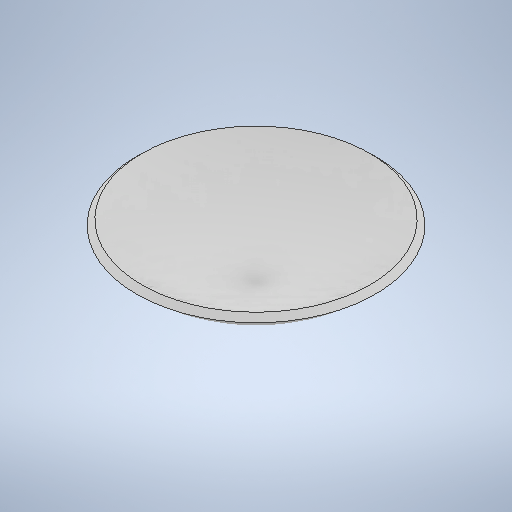
# Autodesk Inventor part: Front Shield Structure
Saved by Autodesk Inventor 2026.2 (Build 302298000, 298)
## iProperties
Created: 2026-01-18
Part Number: Front Shield Structure
Material: Generic
Document SubType Name: Modeling
Designer: daryu
Density: 1 g/cm^3
Appearance: Default
Author: daryu
Autodesk Inventor part; units mm, degrees
ref_plane "YZ Plane" through (0, 0, 0) normal (1, 0, 0) x (0, 1, 0)
ref_plane "XZ Plane" through (0, 0, 0) normal (0, 1, 0) x (-1, 0, 0)
ref_plane "XY Plane" through (0, 0, 0) normal (0, 0, 1) x (1, 0, 0)
sketch "Sketch1" plane through (0, 0, 0) normal (0, 0, 1) x (1, 0, 0)
  arc A0 (-31.4158, 15.3864) -> (0, 0) centre (10.1768, 60.5444) ccw
  arc A1 (-31.4158, 15.3864) -> (0, 0) centre (10.1768, 60.5444) ccw
  line L0 (-31.4158, 15.3864) -> (-29.9776, 16.7762)
  line L1 (0, 0) -> (0, 2)
  arc A2 (-29.9776, 16.7762) -> (0, 2) centre (9.8435, 59.7672) ccw
  line L2 (0, 0) -> (0, 4.1042)
  dimension "d0" = 2
  dimension "d1" = 58.5999
  dimension "d2" = 31.4158
  dimension "d3" = 61.3938
  dimension "d4" = 4.1042
  dimension "d5" = 29.9776
  constraints: 7 point on circle, 6 end point, 3 centre point, 2 vertical, 1 equal length
  measures "d0" distance of L0.start L0.end
  measures "d1" radius of A2
  measures "d2" horizontal distance of L2.start L0.start
  measures "d3" radius of A0
  measures "d4" distance of L2.start L2.end
  measures "d5" horizontal distance of L1.end L0.end
revolve "Revolution1" add sketch "Sketch1" angle 360 about axis through (0, 0, 0) along (0, 1, 0)
sketch "Sketch2" plane through (0, 0, 0) normal (1, 0, 0) x (0, 1, 0)
  arc A0 (16.7762, 29.9776) -> (2, 0) centre (59.7672, -9.8435) ccw projected
  line L0 (6.6004, 14.7987) -> (26.8392, 8.912)
  line L1 (26.8392, 0) -> (26.8392, 8.912)
  line L2 (2, 0) -> (26.8392, 0)
  point P0 (0, 0)
  constraints: 6 end point, 1 horizontal, 1 point on circle, 1 vertical
sketch "Sketch3" plane through (0, 0, 0) normal (1, 0, 0) x (0, 1, 0)
  line L0 (6.6004, 14.7987) -> (6.6004, -14.7987) projected
  line L1 (26.8392, -8.912) -> (26.8392, 8.912) projected
  line L2 (6.6004, 14.7987) -> (26.8392, 8.912)
  line L3 (26.8392, 8.912) -> (29.8656, 8.0317)
  line L4 (29.8656, 8.0317) -> (29.8656, 10.0317)
  line L5 (29.8656, 10.0317) -> (7.4487, 16.552)
  arc A0 (16.7762, 29.9776) -> (6.6004, 14.7987) centre (59.7672, -9.8435) ccw projected
  line L6 (6.6004, 0) -> (10.7627, 0)
  point P0 (0, 0)
  dimension "d9" = 2
  constraints: 4 end point, 1 collinear, 1 vertical
  measures "d9" distance of L3.end L4.end
body "Solid1"
